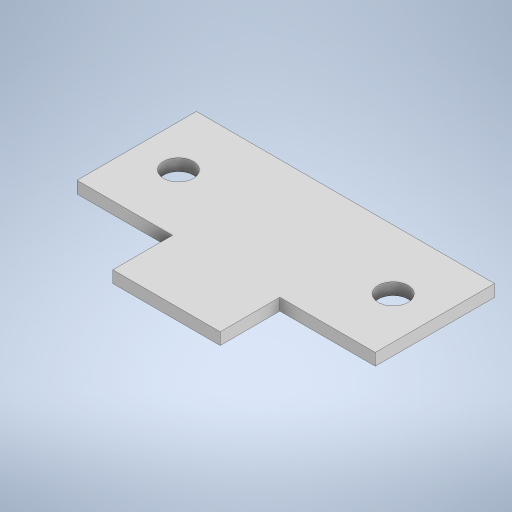
# Autodesk Inventor part: gps_lid
Saved by Autodesk Inventor 2024 (Build 280153000, 153)
## iProperties
Created: 2025-12-27
Part Number: gps_lid
Material: Generic
Document SubType Name: Modeling
Designer: schar
Density: 1 g/cm^3
Appearance: Default
Author: schar
Autodesk Inventor part; units mm, degrees
ref_plane "YZ Plane" through (0, 0, 0) normal (1, 0, 0) x (0, 1, 0)
ref_plane "XZ Plane" through (0, 0, 0) normal (0, 1, 0) x (-1, 0, 0)
ref_plane "Work Plane1" through (-25, 9, -10) normal (0, 1, 0) x (1, 0, 0)
sketch "Sketch1" plane through (-25, 9, -10) normal (0, 1, 0) x (1, 0, 0)
  line L0 (0, 0) -> (0, -20) projected
  line L1 (50, -20) -> (50, 0) projected
  line L2 (0, 0) -> (50, 0)
  line L3 (50, 0) -> (50, -20)
  line L4 (50, -20) -> (0, -20)
  line L5 (0, -20) -> (0, 0)
  line L6 (34, -20) -> (34, -30) projected
  line L7 (16, -30) -> (34, -30) projected
  line L8 (34, -20) -> (16, -20)
  line L9 (16, -20) -> (16, -30)
  line L10 (16, -30) -> (34, -30)
  line L11 (34, -30) -> (34, -20)
  circle A0 centre (7, -10) radius 2.5 projected
  circle A1 centre (7, -10) radius 2.5
  circle A2 centre (43, -10) radius 2.5 projected
  circle A3 centre (43, -10) radius 2.5
  point P0 (25, -10)
  constraints: 16 end point, 4 parallel, 2 centre point, 2 coincident, 2 horizontal, 2 perpendicular
extrude "Extrusion1" add sketch "Sketch1" along normal blind 2
body "Solid1"
